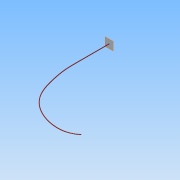
# Autodesk Inventor part: филамент красный
Saved by Autodesk Inventor 2017 (Build 210142000, 142)
## iProperties
Part Number: филамент красный
Material: Типовые
Document SubType Name: Modeling
Designer: Max
Mass: 0.979729 g
Surface Area: 21.8218 cm^2
Volume: 0.979729 cm^3
Density: 1 g/cm^3
Appearance: Светло-красный
Author: Max
Autodesk Inventor part; units mm, degrees
ref_plane "YZ Plane" through (0, 0, 0) normal (1, 0, 0) x (0, 1, 0)
ref_plane "XZ Plane" through (0, 0, 0) normal (0, 1, 0) x (-1, 0, 0)
ref_plane "XY Plane" through (0, 0, 0) normal (0, 0, 1) x (1, 0, 0)
sketch "Эскиз1" plane through (0, 0, 0) normal (0, 0, 1) x (1, 0, 0)
  line L0 (4.5394, -14.081) -> (4.5394, -90.9085)
  line L1 (4.5394, -90.9085) -> (4.5394, -118.3284) construction
  line L2 (4.5394, -118.3284) -> (4.5394, -147.3964) construction
  line L3 (4.5394, -147.3964) -> (12.2069, -179.0249) construction
  line L4 (12.2069, -179.0249) -> (32.6536, -230.4611) construction
  line L5 (32.6536, -230.4611) -> (81.9235, -278.2319) construction
  line L6 (81.9235, -278.2319) -> (132.0554, -286.4431) construction
  line L7 (132.0554, -286.4431) -> (163.9598, -286.4431) construction
  line L8 (163.9598, -286.4431) -> (181.8507, -278.2319) construction
  spline S0 degree 4 poles (4.5394, -90.9085) (4.5394, -118.3284) (4.5394, -147.3964) (12.2069, -179.0249) (32.6536, -230.4611) (81.9235, -278.2319) (132.0554, -286.4431) (163.9598, -286.4431) (181.8507, -278.2319) knots 1 1 1 1 1 2 3 4 5 6 6 6 6 6
  point P0 (0, 0)
  constraints: 2 end point, 2 point on line, 1 vertical, 3 other
ref_plane "РабПлоскость1" through (4.5394, -14.081, 0) normal (0, -1, 0) x (1, 0, 0)
sketch "Эскиз2" plane through (4.5394, -14.081, 0) normal (0, -1, 0) x (1, 0, 0)
  circle A0 centre (0, 0) radius 0.9
  point P0 (-4.5394, 0)
  dimension "d0" = 1.8
  constraints: 1 centre point
  measures "d0" diameter of A0
sweep "Сдвиг1" add profiles "Эскиз2" path "Эскиз1"
